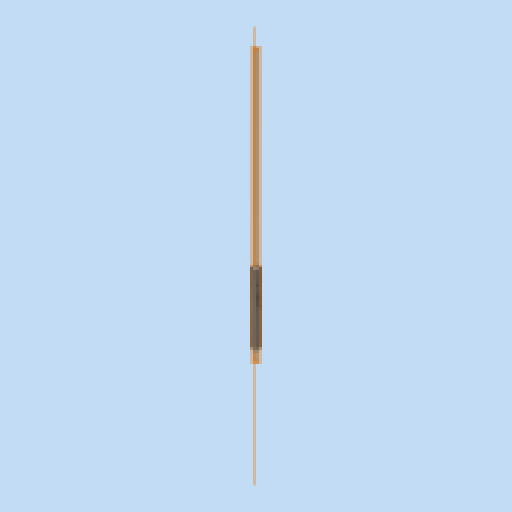
# Autodesk Inventor part: 20x20mmx150mm alminum profile
Saved by Autodesk Inventor 2026.1 (Build 301233000, 233)
## iProperties
Created: 2025-01-21
Part Number: 20x20mmx150mm alminum profile
Material: Aluminum 6061
Document SubType Name: Modeling
Designer: Cupri
Density: 2.7 g/cm^3
Appearance: Aluminum - Flat
Mass: 43.5843 g
Surface Area: 190.944 cm^2
Volume: 16.1423 cm^3
Sending System: Autodesk Translation Framework v13.20.0.188
Preprocessor: ST-DEVELOPER v20
Title: 20x20mmx150mm alminum profile.step
Autodesk Inventor part; units mm, degrees
ref_plane "YZ Plane" through (0, 0, 0) normal (1, 0, 0) x (0, 1, 0)
ref_plane "XZ Plane" through (0, 0, 0) normal (0, 1, 0) x (-1, 0, 0)
ref_plane "Work Plane1" through (-2.7515, 150, 3.6) normal (0, 1, 0) x (1, 0, 0)
sketch "Sketch1" plane through (-2.7515, 150, 3.6) normal (0, 1, 0) x (1, 0, 0)
  arc A0 (-6.7485, 13.6) -> (-7.2485, 13.1) centre (-6.7485, 13.1) ccw projected
  line L0 (-7.2485, 13.1) -> (-7.2485, 8.1) projected
  line L1 (-7.2485, 8.1) -> (-5.7485, 6.6) projected
  line L2 (-5.7485, 6.6) -> (-5.7485, 9.8) projected
  line L3 (-5.7485, 9.8) -> (-4.2971, 9.8) projected
  line L4 (-4.2971, 9.8) -> (-0.8485, 6.3515) projected
  line L5 (-0.8485, 6.3515) -> (-0.8485, 0.8485) projected
  line L6 (-0.8485, 0.8485) -> (-4.2971, -2.6) projected
  line L7 (-4.2971, -2.6) -> (-5.7485, -2.6) projected
  line L8 (-5.7485, -2.6) -> (-5.7485, 0.6) projected
  line L9 (-5.7485, 0.6) -> (-7.2485, -0.9) projected
  line L10 (-7.2485, -0.9) -> (-7.2485, -5.9) projected
  arc A1 (-7.2485, -5.9) -> (-6.7485, -6.4) centre (-6.7485, -5.9) ccw projected
  line L11 (-6.7485, -6.4) -> (-1.7485, -6.4) projected
  line L12 (-1.7485, -6.4) -> (-0.2485, -4.9) projected
  line L13 (-0.2485, -4.9) -> (-3.4485, -4.9) projected
  line L14 (-3.4485, -4.9) -> (-3.4485, -3.4485) projected
  line L15 (-3.4485, -3.4485) -> (0, 0) projected
  line L16 (0, 0) -> (5.5029, 0) projected
  line L17 (5.5029, 0) -> (8.9515, -3.4485) projected
  line L18 (8.9515, -3.4485) -> (8.9515, -4.9) projected
  line L19 (8.9515, -4.9) -> (5.7515, -4.9) projected
  line L20 (5.7515, -4.9) -> (7.2515, -6.4) projected
  line L21 (7.2515, -6.4) -> (12.2515, -6.4) projected
  arc A2 (12.2515, -6.4) -> (12.7515, -5.9) centre (12.2515, -5.9) ccw projected
  line L22 (12.7515, -5.9) -> (12.7515, -0.9) projected
  line L23 (12.7515, -0.9) -> (11.2515, 0.6) projected
  line L24 (11.2515, 0.6) -> (11.2515, -2.6) projected
  line L25 (11.2515, -2.6) -> (9.8, -2.6) projected
  line L26 (9.8, -2.6) -> (6.3515, 0.8485) projected
  line L27 (6.3515, 0.8485) -> (6.3515, 6.3515) projected
  line L28 (6.3515, 6.3515) -> (9.8, 9.8) projected
  line L29 (9.8, 9.8) -> (11.2515, 9.8) projected
  line L30 (11.2515, 9.8) -> (11.2515, 6.6) projected
  line L31 (11.2515, 6.6) -> (12.7515, 8.1) projected
  line L32 (12.7515, 8.1) -> (12.7515, 13.1) projected
  arc A3 (12.7515, 13.1) -> (12.2515, 13.6) centre (12.2515, 13.1) ccw projected
  line L33 (12.2515, 13.6) -> (7.2515, 13.6) projected
  line L34 (7.2515, 13.6) -> (5.7515, 12.1) projected
  line L35 (5.7515, 12.1) -> (8.9515, 12.1) projected
  line L36 (8.9515, 12.1) -> (8.9515, 10.6485) projected
  line L37 (8.9515, 10.6485) -> (5.5029, 7.2) projected
  line L38 (5.5029, 7.2) -> (0, 7.2) projected
  line L39 (0, 7.2) -> (-3.4485, 10.6485) projected
  line L40 (-3.4485, 10.6485) -> (-3.4485, 12.1) projected
  line L41 (-3.4485, 12.1) -> (-0.2485, 12.1) projected
  line L42 (-0.2485, 12.1) -> (-1.7485, 13.6) projected
  line L43 (-1.7485, 13.6) -> (-6.7485, 13.6) projected
  circle A4 centre (2.7515, 3.6) radius 2 projected
extrude "Extrusion1" add sketch "Sketch1" along normal blind 230
ref_plane "Work Plane2" through (0, 150, -9.5) normal (1, 0, 0) x (0, 0, -1)
ref_plane "Work Plane3" through (-4.5, 150, 0) normal (0, 0, 1) x (1, 0, 0)
body "Solid2"
